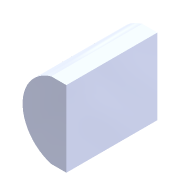
# Autodesk Inventor part: 00_Thorlabs_LJ1878L1-A-Step
Saved by Autodesk Inventor 2022 (Build 260153000, 153)
## iProperties
Created: 2010-04-22
Part Number: 00_Thorlabs_LJ1878L1-A-Step
Material: Generisch
Description: STEP AP214
Document SubType Name: Modeling
Designer: diederichbenedict
Density: 1 g/cm^3
Appearance: Vorgabe
Title: 5516-E0W.STEP
Revision Number: ANY
Sending System: SolidWorks 2009
Preprocessor: SwSTEP 2.0
Autodesk Inventor part; units mm, degrees
ref_plane "YZ Plane" through (0, 0, 0) normal (1, 0, 0) x (0, 1, 0)
ref_plane "XZ Plane" through (0, 0, 0) normal (0, 1, 0) x (-1, 0, 0)
ref_plane "XY Plane" through (0, 0, 0) normal (0, 0, 1) x (1, 0, 0)
sketch "Skizze1" plane through (0, 0, 0) normal (0, 0, 1) x (1, 0, 0)
  line L0 (0, 0) -> (-2, 0)
  line L1 (-2, 0) -> (-2, 10)
  line L2 (-2, 10) -> (0, 10)
  line L3 (0, 10) -> (0, 0)
  arc A0 (-2, 10) -> (-2, 0) centre (-0.5717, 5) ccw
  dimension "d0" = 2
  dimension "d1" = 10
  dimension "d2" = 5.2
  constraints: 8 end point, 2 parallel, 2 point on circle, 1 centre point, 1 horizontal, 1 perpendicular
  measures "d0" distance of L1.end L2.end
  measures "d1" distance of L0.end L1.end
  measures "d2" radius of A0
extrude "Extrusion1" add sketch "Skizze1" along normal blind 12
ref_plane "Arbeitsebene1" through (-2, 5, 0) normal (0, -1, 0) x (1, 0, 0)
ref_plane "Arbeitsebene2" through (0, 0, 6) normal (0, 0, -1) x (-1, 0, 0)
